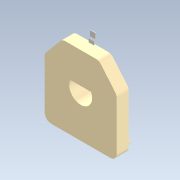
# Autodesk Inventor part: potentiometer_bourns_3382_12mm
Saved by Autodesk Inventor 2020.2 (Build 242310000, 310)
## iProperties
Created: 2020-04-25
Part Number: potentiometer_bourns_3382_12mm
Material: Generic
Document SubType Name: Modeling
Designer: Bardo91
Density: 1 g/cm^3
Appearance: Default
Author: Bardo91
Autodesk Inventor part; units mm, degrees
ref_plane "YZ Plane" through (0, 0, 0) normal (1, 0, 0) x (0, 1, 0)
ref_plane "XZ Plane" through (0, 0, 0) normal (0, 1, 0) x (-1, 0, 0)
ref_plane "XY Plane" through (0, 0, 0) normal (0, 0, 1) x (1, 0, 0)
sketch "Sketch1" plane through (0, 0, 0) normal (0, 0, 1) x (1, 0, 0)
  line L0 (-2.3351, 6) -> (2.3351, 6)
  line L1 (5.5, 2.42) -> (5.5, -5)
  line L2 (4.5, -6) -> (-4.5, -6)
  line L3 (-5.5, -5) -> (-5.5, 2.42)
  line L4 (0, 6) -> (0, -6)
  line L5 (0, -6) -> (0, 0.5)
  circle A0 centre (0, 0.5) radius 1.75
  line L6 (0, 2.25) -> (0, 1.25)
  line L7 (0, 1.25) -> (1.5811, 1.25)
  line L8 (0, 1.25) -> (-1.5811, 1.25)
  line L9 (-5.266, 3.0628) -> (-3.1012, 5.6428)
  line L10 (5.266, 3.0628) -> (3.1012, 5.6428)
  arc A1 (-5.266, 3.0628) -> (-5.5, 2.42) centre (-4.5, 2.42) ccw
  arc A2 (-2.3351, 6) -> (-3.1012, 5.6428) centre (-2.3351, 5) ccw
  arc A3 (3.1012, 5.6428) -> (2.3351, 6) centre (2.3351, 5) ccw
  arc A4 (5.5, 2.42) -> (5.266, 3.0628) centre (4.5, 2.42) ccw
  arc A5 (4.5, -6) -> (5.5, -5) centre (4.5, -5) ccw
  arc A6 (-5.5, -5) -> (-4.5, -6) centre (-4.5, -5) ccw
  point P0 (0, 0)
  point P1 (5.5, -6)
  point P2 (-5.5, -6)
  point P3 (0, 0)
  dimension "d0" = 11
  dimension "d2" = 6.5
  dimension "d3" = 3.5
  dimension "d4" = 1
  dimension "d9" = 1
  dimension "d10" = 12
  dimension "d11" = 3.58
  dimension "d12" = 3.58
  dimension "d13" = 40
  dimension "d14" = 40
  constraints: 22 end point, 15 point on circle, 12 tangent, 8 point on line, 7 centre point, 5 equal radius, 3 midpoint, 2 coincident, 2 parallel, 2 perpendicular, 1 horizontal
  measures "d0" distance of point (5.5, -6) point (-5.5, -6)
  measures "d2" distance of L4.end L5.end
  measures "d3" diameter of A0
  measures "d4" distance of L6.start L6.end
  measures "d9" radius of A1
  measures "d10" distance between parallel lines of L2 L0
  measures "d11" distance from line of L0 A4.centre
  measures "d12" distance from line of L0 A1.centre
  measures "d13" angle of L3 L9
  measures "d14" angle of L1 L10
extrude "Extrusion1" add sketch "Sketch1" along normal blind 1.85 contours L0 L4 A0 L2 A6 L3 A1 L9 A2 | L0 A3 L10 A4 L1 A5 L2 L4 A0 | A0 L7 L4 | L4 L8 A0 picked at (0.9848, 1.3616) picked at (-0.9848, 1.3616)
sketch "Sketch2" plane through (0, 0, 0) normal (0, 0, -1) x (-1, 0, 0)
  arc A0 (-5.5, -5) -> (-4.5, -6) centre (-4.5, -5) ccw projected
  circle A1 centre (-4.5, -5) radius 0.5
  arc A2 (4.5, -6) -> (5.5, -5) centre (4.5, -5) ccw projected
  circle A3 centre (4.5, -5) radius 0.5
  point P0 (0, 0)
  dimension "d17" = 1
  dimension "d18" = 1
  constraints: 2 centre point, 2 coincident
  measures "d17" diameter of A1
  measures "d18" diameter of A3
extrude "Extrusion2" add sketch "Sketch2" along normal blind 1
fillet "Fillet1" radius 0.5 2 edges at (5, -5, -1) (-4, -5, -1)
sketch "Sketch3" plane through (0, 0, 0) normal (0, 0, -1) x (-1, 0, 0)
  arc A0 (-1.5811, 1.25) -> (1.5811, 1.25) centre (0, 0.5) ccw projected
  arc A1 (-1.5811, 1.25) -> (1.5811, 1.25) centre (0, 0.5) ccw
  line L0 (1.5811, 1.25) -> (-1.5811, 1.25) projected
  line L1 (1.5811, 1.25) -> (-1.5811, 1.25)
  arc A2 (-1.8708, 1.75) -> (1.8708, 1.75) centre (0, 0.5) ccw
  line L2 (-1.8708, 1.75) -> (1.8708, 1.75)
  point P0 (0, 0)
  dimension "d22" = 0.5
  constraints: 4 end point, 4 point on circle, 2 centre point, 1 coincident, 1 collinear, 1 other
  measures "d22" distance between parallel lines of L0 L2
extrude "Extrusion3" add sketch "Sketch3" along normal blind 1
sketch "Sketch4" plane through (0, 0, 0) normal (1, 0, 0) x (0, 1, 0)
  line L0 (-6, 0) -> (-6, 1.85) projected
  line L1 (-6, 0) -> (-6, 0.1)
  line L2 (-7.5, -0.1) -> (-7.5, 0)
  line L3 (-7.5, 0) -> (-6.7052, 0)
  line L4 (-6.7052, 0) -> (-6.5, 0.2203)
  line L5 (-6.5, 0.2203) -> (-6, 0.2203)
  line L6 (-6, 0.1) -> (-6.4138, 0.1)
  line L7 (-6.4138, 0.1) -> (-6.6026, -0.1)
  line L8 (-6.6026, -0.1) -> (-7.5, -0.1)
  point P0 (0, 0)
  dimension "d25" = 0.1
  dimension "d29" = 0.1
  constraints: 16 end point, 2 perpendicular, 2 point on line, 1 horizontal
  measures "d25" distance of L0.start L1.end
  measures "d29" distance of L2.start L2.end
extrude "Extrusion4" add sketch "Sketch4" against normal mid plane 0.8
mirror "Mirror1" about plane through (0, 0, 0) normal (0, 1, 0) of "Extrusion4"
pattern_linear "Rectangular Pattern1" count 2 spacing 2 along (1, 0, 0) of "Extrusion4"
pattern_linear "Rectangular Pattern2" count 2 spacing 2 along (-1, 0, 0) of "Extrusion4"
body "Solid1"
